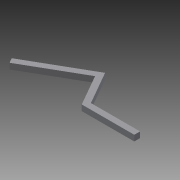
# Autodesk Inventor part: bar 3
Saved by Autodesk Inventor 2013 (Build 170138000, 138)
## iProperties
Created: 2013-03-02
Part Number: bar 3
Material: Generic
Document SubType Name: Modeling
Designer: Arpan
Density: 1 g/cm^3
Author: Arpan
Autodesk Inventor part; units mm, degrees
ref_plane "YZ Plane" through (0, 0, 0) normal (1, 0, 0) x (0, 1, 0)
ref_plane "XZ Plane" through (0, 0, 0) normal (0, 1, 0) x (-1, 0, 0)
ref_plane "XY Plane" through (0, 0, 0) normal (0, 0, 1) x (1, 0, 0)
sketch "Sketch1" plane through (0, 0, 0) normal (0, 1, 0) x (-1, 0, 0)
  line L0 (-660.4, 0) -> (-660.4, 25.4)
  line L1 (-113.1604, 25.4) -> (-351.652, -111.264)
  line L2 (-351.652, -111.264) -> (-415.4102, 0)
  line L3 (-444.6849, 0) -> (-660.4, 0)
  line L4 (-660.4, 0) -> (-660.4, 25.4)
  line L5 (-660.4, 25.4) -> (-429.9653, 25.4)
  line L6 (-429.9653, 25.4) -> (-415.4102, 0)
  line L7 (-113.1604, 25.4) -> (-100.5318, 3.3619)
  line L8 (-100.5318, 3.3619) -> (-361.0615, -145.9308)
  line L9 (-361.0615, -145.9308) -> (-444.6849, 0)
  line L10 (-660.4, 0) -> (-660.4, 25.4)
  line L11 (-113.1604, 25.4) -> (-351.652, -111.264)
  line L12 (-351.652, -111.264) -> (-415.4102, 0)
  line L13 (-444.6849, 0) -> (-660.4, 0)
  line L14 (-660.4, 0) -> (-660.4, 25.4)
  line L15 (-660.4, 25.4) -> (-429.9653, 25.4)
  line L16 (-429.9653, 25.4) -> (-415.4102, 0)
  line L17 (-113.1604, 25.4) -> (-100.5318, 3.3619)
  line L18 (-100.5318, 3.3619) -> (-361.0615, -145.9308)
  line L19 (-361.0615, -145.9308) -> (-444.6849, 0)
  point P0 (0, 0)
  point P1 (-113.1604, 0)
  point P2 (-113.1604, 0)
  dimension "d0" = 25.4
  dimension "d1" = 25.4
  dimension "d2" = 25.4
  dimension "d3" = 25.4
  dimension "d4" = 25.4
  dimension "d5" = 25.4
  constraints: 40 end point, 6 perpendicular, 2 parallel
  measures "d0" distance of L1.start point (-113.16, 0)
  measures "d1" distance of L1.start L7.end
  measures "d2" distance between parallel lines of L2 L9
  measures "d3" distance of L11.start point (-113.16, 0)
  measures "d4" distance of L11.start L17.end
  measures "d5" distance between parallel lines of L12 L19
extrude "Extrusion1" add sketch "Sketch1" along normal blind 25.4
body "Solid1"
